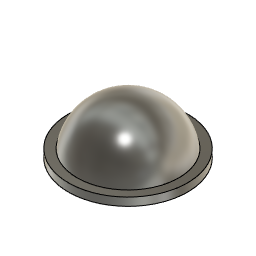
POP_endcap_derated (Autodesk Fusion 360 design; units mm, degrees)
Autodesk Fusion 360 part; units mm, degrees
sketch "Sketch1" plane through (0, 0, 0) normal (0, 1, 0) x (1, 0, 0)
  line L0 (-36, 0) -> (40, 0) construction
  arc A0 (-32, 0) -> (0, -32) centre (0, 0) ccw
  arc A1 (-25.65, 0) -> (0, -25.65) centre (0, 0) ccw
  line L1 (0, -32) -> (0, -25.65)
  line L2 (-25.65, 0) -> (-32, 0)
  dimension "d3" = 25.65
  dimension "d4" = 32
  constraint coincident A0.centre A1.centre
  constraint horizontal L0
  constraint coincident L0 A0.start
  constraint coincident L0 A1.start
  measures "d3" radius of A1
  measures "d4" radius of A0
revolve "Revolve1" add sketch "Sketch1" angle 360 about axis through (0, 0, 1.75) along (0, 0, 1)
sketch "Sketch3" plane through (0, 0, 0) normal (0, 0, -1) x (1, 0, 0)
  circle A0 centre (0, 0) radius 32
  circle A1 centre (0, 0) radius 37
  circle A2 centre (0, 0) radius 25.65
  circle A3 centre (0, 0) radius 25.65
  dimension "d10" = 74
  constraint coincident A0.centre A1.centre
  constraint concentric A1 A3
  measures "d10" diameter of A1
extrude "Extrude2" add sketch "Sketch3" against normal blind 5 contours A0 | A1
sketch "Sketch2" plane through (0, 0, 0) normal (0, 0, -1) x (1, 0, 0)
  circle A0 centre (0, 0) radius 28.37
  circle A1 centre (0, 0) radius 32.05
  circle A2 centre (0, 0) radius 37
  circle A3 centre (0, 0) radius 25.65
  dimension "d6" = 56.74
  dimension "d7" = 64.1
  constraint coincident A0.centre A1.centre
  measures "d6" diameter of A0
  measures "d7" diameter of A1
extrude "Extrude1" cut sketch "Sketch2" against normal blind 2.794 contours A1
fillet "Fillet1" radius 0.1 2 edges at (-26.4501, 10.259, 2.794) (-29.8811, -11.5898, 2.794)
